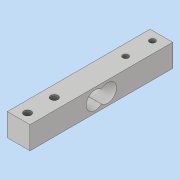
# Autodesk Inventor part: LoadCell
Saved by Autodesk Inventor 2018 (Build 220112000, 112)
## iProperties
Created: 2020-10-04
Part Number: LoadCell
Material: Generisch
Document SubType Name: Modeling
Designer: marce
Density: 1 g/cm^3
Appearance: Vorgabe
Author: marce
Autodesk Inventor part; units mm, degrees
ref_plane "YZ Plane" through (0, 0, 0) normal (1, 0, 0) x (0, 1, 0)
ref_plane "XZ Plane" through (0, 0, 0) normal (0, 1, 0) x (-1, 0, 0)
ref_plane "XY Plane" through (0, 0, 0) normal (0, 0, 1) x (1, 0, 0)
sketch "Skizze1" plane through (0, 0, 0) normal (0, 0, 1) x (1, 0, 0)
  line L0 (0, 0) -> (12.7, 0)
  line L1 (12.7, 0) -> (12.7, 80)
  line L2 (12.7, 80) -> (0, 80)
  line L3 (0, 80) -> (0, 0)
  dimension "d0" = 12.7
  dimension "d1" = 80
  constraints: 8 end point, 2 parallel, 1 horizontal, 1 perpendicular
  measures "d0" distance of L2.end L1.end
  measures "d1" distance of L1.end L0.end
extrude "Extrusion1" add sketch "Skizze1" along normal blind 12.7
sketch "Skizze2" plane through (0, 0, 12.7) normal (0, 0, 1) x (1, 0, 0)
  line L0 (0, 0) -> (12.7, 0) projected
  line L1 (6.35, 0) -> (5, 0)
  line L2 (5, 0) -> (5, 5)
  line L3 (5, 5) -> (6.35, 5)
  line L4 (6.35, 5) -> (6.35, 0)
  line L5 (6.35, 5) -> (2, 5)
  line L6 (2, 5) -> (2, 20)
  line L7 (2, 20) -> (6.35, 20)
  line L8 (6.35, 20) -> (6.35, 5)
  dimension "d4" = 5
  dimension "d5" = 15
  constraints: 16 end point, 4 parallel, 2 horizontal, 2 perpendicular, 1 midpoint
  measures "d4" distance of L1.end L2.end
  measures "d5" distance of L5.end L6.end
hole "Bohrung1" at (6.35, 5, 12.7) at (6.35, 20, 12.7) direction (0, 0, -1) diameter 4.134 end through all thread size "M5x0.8" class "6H" standard "ISO Metric profile"
sketch "Skizze3" plane through (0, 0, 12.7) normal (0, 0, 1) x (1, 0, 0)
  line L0 (12.7, 80) -> (0, 80) projected
  line L1 (6.35, 80) -> (4, 80)
  line L2 (4, 80) -> (4, 75)
  line L3 (4, 75) -> (6.35, 75)
  line L4 (6.35, 75) -> (6.35, 80)
  line L5 (6.35, 75) -> (4, 75)
  line L6 (4, 75) -> (4, 60)
  line L7 (4, 60) -> (6.35, 60)
  line L8 (6.35, 60) -> (6.35, 75)
  point P0 (0, 0)
  dimension "d13" = 5
  dimension "d14" = 15
  constraints: 16 end point, 4 parallel, 2 horizontal, 2 perpendicular, 1 midpoint, 1 point on line
  measures "d13" distance of L2.end L1.end
  measures "d14" distance of L6.end L5.end
hole "Bohrung2" at (6.35, 60, 12.7) at (6.35, 75, 12.7) direction (0, 0, -1) diameter 3.242 end through all thread size "M4x0.7" class "6H" standard "ISO Metric profile"
sketch "Skizze4" plane through (12.7, 0, 0) normal (1, 0, 0) x (0, 0, -1)
  line L0 (0, 0) -> (-12.7, 0) projected
  line L1 (-12.7, 0) -> (-12.7, 80) projected
  line L2 (-6.35, 0) -> (-12.7, 0)
  line L3 (-12.7, 0) -> (-12.7, 40)
  line L4 (-12.7, 40) -> (-6.35, 40)
  line L5 (-6.35, 40) -> (-6.35, 0)
  line L6 (-6.35, 36.5) -> (-6.35, 43.5)
  line L7 (-6.35, 43.5) -> (-6.35, 36.5)
  circle A0 centre (-6.35, 36.5) radius 5
  circle A1 centre (-6.35, 43.5) radius 5
  point P0 (-6.35, 40)
  dimension "d22" = 7
  dimension "d23" = 10
  dimension "d24" = 10
  constraints: 12 end point, 5 coincident, 4 midpoint, 3 equal length, 2 centre point, 1 horizontal, 1 perpendicular, 1 point on line, 1 vertical, 4 other
  measures "d22" distance of L6.end L6.start
  measures "d23" diameter of A0
  measures "d24" diameter of A1
extrude "Extrusion2" cut sketch "Skizze4" against normal through all contours A0 A1 L5 | L5 A1 A0 | A0 L6 L4 | A1 A0 | L4 L5 A1 | L5 L6 A0 A1
equation "\"d24\" = d23"
